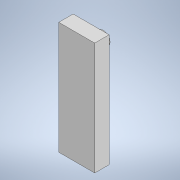
# Autodesk Inventor part: regulararm
Saved by Autodesk Inventor 2021.2 (Build 252289000, 289)
## iProperties
Created: 2021-03-03
Part Number: regulararm
Material: Generic
Document SubType Name: Modeling
Designer: zayda
Density: 1 g/cm^3
Appearance: Default
Author: zayda
Autodesk Inventor part; units mm, degrees
ref_plane "YZ Plane" through (0, 0, 0) normal (1, 0, 0) x (0, 1, 0)
ref_plane "XZ Plane" through (0, 0, 0) normal (0, 1, 0) x (-1, 0, 0)
ref_plane "XY Plane" through (0, 0, 0) normal (0, 0, 1) x (1, 0, 0)
sketch "Sketch1" plane through (0, 0, 0) normal (0, 0, 1) x (1, 0, 0)
  line L0 (0, 0) -> (25.4, 0)
  line L1 (25.4, 0) -> (25.4, 76.2)
  line L2 (25.4, 76.2) -> (0, 76.2)
  line L3 (0, 76.2) -> (0, 0)
  dimension "d0" = 25.4
  dimension "d1" = 76.2
  constraints: 8 end point, 2 parallel, 1 horizontal, 1 perpendicular
  measures "d0" distance of L2.end L1.end
  measures "d1" distance of L1.end L0.end
extrude "Extrusion1" add sketch "Sketch1" along normal blind 10.16
sketch "Sketch3" plane through (0, 0, 0) normal (0, -1, 0) x (1, 0, 0)
  line L0 (25.4, 10.16) -> (0, 10.16) projected
  line L1 (25.4, 0) -> (0, 0) projected
  line L2 (0, 10.16) -> (25.4, 10.16)
  line L3 (25.4, 10.16) -> (25.4, 0)
  line L4 (25.4, 0) -> (0, 0)
  line L5 (0, 0) -> (0, 10.16)
  constraints: 8 end point, 2 parallel, 1 horizontal, 1 perpendicular
extrude "Extrusion3" add sketch "Sketch3" along normal blind 3.302
sketch "Sketch4" plane through (0, 0, 0) normal (0, 0, -1) x (-1, 0, 0)
  line L0 (-25.4, 76.2) -> (0, 76.2) projected
  circle A0 centre (-12.7, 63.5) radius 1.905
  circle A1 centre (-12.7, 63.5) radius 4.826
  point P0 (0, 0)
  dimension "d9" = 3.81
  dimension "d10" = 9.652
  constraints: 2 centre point, 1 coincident
  measures "d9" diameter of A0
  measures "d10" diameter of A1
extrude "Extrusion4" add sketch "Sketch4" along normal blind 6.985 contours A0
extrude "Extrusion5" add sketch "Sketch4" along normal blind 8.5725
body "Solid1"
